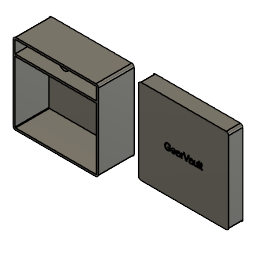
GearVault_Mini (Autodesk Fusion 360 design; units mm, degrees)
part number: 2026-09-08-22-04-46-192
Autodesk Fusion 360 part; units mm, degrees
sketch "Sketch1" plane through (0, 0, 0) normal (0, 0, 1) x (1, 0, 0)
  line L0 (-34.5, -32.5) -> (34.5, -32.5)
  line L1 (34.5, -32.5) -> (34.5, 32.5)
  line L2 (34.5, 32.5) -> (-34.5, 32.5)
  line L3 (-34.5, 32.5) -> (-34.5, -32.5)
extrude "Extrude1" add sketch "Sketch1" along normal blind 29 makes body 1
fillet "Fillet1" radius 2 4 edges at (-34.5, 32.5, 14.5) (34.5, 32.5, 14.5) (34.5, -32.5, 14.5) (-34.5, -32.5, 14.5) on bodies 1
shell "Shell1" thickness 1.6 removed faces 1 at (-10.8333, -10.8333, 29) on bodies 1
sketch "Sketch2" plane through (0, 0, 0) normal (0, 0, 1) x (1, 0, 0)
  line L0 (-32.9, 19.1) -> (32.9, 19.1)
  line L1 (32.9, 19.1) -> (32.9, 20.7)
  line L2 (32.9, 20.7) -> (-32.9, 20.7)
  line L3 (-32.9, 20.7) -> (-32.9, 19.1)
extrude "Extrude2" add sketch "Sketch2" along normal blind 29 bodies 1
sketch "Sketch3" plane through (0, 0, 0) normal (0, 0, 1) x (1, 0, 0)
  circle A0 centre (0, 25.8) radius 4
extrude "Extrude3" add sketch "Sketch3" along normal blind 22 bodies 1
sketch "Sketch4" plane through (0, 0, 0) normal (0, 0, 1) x (1, 0, 0)
  line L0 (49.5, -34.4) -> (122.3, -34.4)
  line L1 (122.3, -34.4) -> (122.3, 34.4)
  line L2 (122.3, 34.4) -> (49.5, 34.4)
  line L3 (49.5, 34.4) -> (49.5, -34.4)
sketch "Sketch6" plane through (0, 0, 0) normal (0, 0, 1) x (1, 0, 0)
  line L0 (49.5, -34.4) -> (122.3, -34.4)
  line L1 (122.3, -34.4) -> (122.3, 34.4)
  line L2 (122.3, 34.4) -> (49.5, 34.4)
  line L3 (49.5, 34.4) -> (49.5, -34.4)
extrude "Extrude6" add sketch "Sketch6" along normal blind 11.6 separate body makes body 2
fillet "Fillet3" radius 2 4 edges at (49.5, 34.4, 5.8) (122.3, 34.4, 5.8) (122.3, -34.4, 5.8) (49.5, -34.4, 5.8) on bodies 2
shell "Shell3" thickness 1.6 removed faces 1 at (74.4333, -11.4667, 0) on bodies 2
sketch "Sketch9" plane through (0, 0, 11.6) normal (0, 0, 1) x (1, 0, 0)
  arc A0 (49.5, -32.4) -> (51.5, -34.4) centre (51.5, -32.4) ccw
  line L0 (51.5, -34.4) -> (120.3, -34.4)
  arc A1 (120.3, -34.4) -> (122.3, -32.4) centre (120.3, -32.4) ccw
  line L1 (122.3, -32.4) -> (122.3, 32.4)
  arc A2 (122.3, 32.4) -> (120.3, 34.4) centre (120.3, 32.4) ccw
  line L2 (120.3, 34.4) -> (51.5, 34.4)
  arc A3 (51.5, 34.4) -> (49.5, 32.4) centre (51.5, 32.4) ccw
  line L3 (49.5, 32.4) -> (49.5, -32.4)
  line L4 (73.1527, -0.5389) -> (73.1527, 0.0477)
  line L5 (73.1527, 0.0477) -> (75.2707, 0.0512)
  line L6 (75.2707, 0.0512) -> (75.2707, -1.8042)
  spline S0 degree 2 poles (75.2707, -1.8042) (74.783, -2.193) (74.2646, -2.3892) knots 0 0 0 1 1 1
  spline S1 degree 2 poles (74.2646, -2.3892) (73.7462, -2.5853) (73.2005, -2.5853) knots 0 0 0 1 1 1
  spline S2 degree 2 poles (73.2005, -2.5853) (72.4638, -2.5853) (71.8618, -2.2698) knots 0 0 0 1 1 1
  spline S3 degree 2 poles (71.8618, -2.2698) (71.2598, -1.9543) (70.9529, -1.3574) knots 0 0 0 1 1 1
  spline S4 degree 2 poles (70.9529, -1.3574) (70.6459, -0.7606) (70.6459, -0.0239) knots 0 0 0 1 1 1
  spline S5 degree 2 poles (70.6459, -0.0239) (70.6459, 0.706) (70.9512, 1.3387) knots 0 0 0 1 1 1
  spline S6 degree 2 poles (70.9512, 1.3387) (71.2564, 1.9714) (71.8294, 2.2783) knots 0 0 0 1 1 1
  spline S7 degree 2 poles (71.8294, 2.2783) (72.4024, 2.5853) (73.1493, 2.5853) knots 0 0 0 1 1 1
  spline S8 degree 2 poles (73.1493, 2.5853) (73.6916, 2.5853) (74.1299, 2.4096) knots 0 0 0 1 1 1
  spline S9 degree 2 poles (74.1299, 2.4096) (74.5681, 2.234) (74.8171, 1.9202) knots 0 0 0 1 1 1
  spline S10 degree 2 poles (74.8171, 1.9202) (75.0661, 1.6064) (75.1957, 1.1016) knots 0 0 0 1 1 1
  line L7 (75.1957, 1.1016) -> (74.5988, 0.9379)
  spline S11 degree 2 poles (74.5988, 0.9379) (74.4863, 1.3199) (74.3192, 1.5382) knots 0 0 0 1 1 1
  spline S12 degree 2 poles (74.3192, 1.5382) (74.152, 1.7565) (73.8417, 1.8878) knots 0 0 0 1 1 1
  spline S13 degree 2 poles (73.8417, 1.8878) (73.5313, 2.0191) (73.1527, 2.0191) knots 0 0 0 1 1 1
  spline S14 degree 2 poles (73.1527, 2.0191) (72.6991, 2.0191) (72.3683, 1.881) knots 0 0 0 1 1 1
  spline S15 degree 2 poles (72.3683, 1.881) (72.0374, 1.7428) (71.8345, 1.5177) knots 0 0 0 1 1 1
  spline S16 degree 2 poles (71.8345, 1.5177) (71.6316, 1.2926) (71.519, 1.0232) knots 0 0 0 1 1 1
  spline S17 degree 2 poles (71.519, 1.0232) (71.328, 0.5593) (71.328, 0.0171) knots 0 0 0 1 1 1
  spline S18 degree 2 poles (71.328, 0.0171) (71.328, -0.6514) (71.5583, -1.1016) knots 0 0 0 1 1 1
  spline S19 degree 2 poles (71.5583, -1.1016) (71.7885, -1.5518) (72.2284, -1.7701) knots 0 0 0 1 1 1
  spline S20 degree 2 poles (72.2284, -1.7701) (72.6684, -1.9884) (73.163, -1.9884) knots 0 0 0 1 1 1
  spline S21 degree 2 poles (73.163, -1.9884) (73.5927, -1.9884) (74.002, -1.823) knots 0 0 0 1 1 1
  spline S22 degree 2 poles (74.002, -1.823) (74.4113, -1.6576) (74.6227, -1.47) knots 0 0 0 1 1 1
  line L8 (74.6227, -1.47) -> (74.6227, -0.5389)
  line L9 (74.6227, -0.5389) -> (73.1527, -0.5389)
  line L10 (78.6473, -1.3336) -> (79.2817, -1.412)
  spline S23 degree 2 poles (79.2817, -1.412) (79.1316, -1.9679) (78.7257, -2.2749) knots 0 0 0 1 1 1
  spline S24 degree 2 poles (78.7257, -2.2749) (78.3199, -2.5819) (77.6889, -2.5819) knots 0 0 0 1 1 1
  spline S25 degree 2 poles (77.6889, -2.5819) (76.8942, -2.5819) (76.4286, -2.0924) knots 0 0 0 1 1 1
  spline S26 degree 2 poles (76.4286, -2.0924) (75.9631, -1.603) (75.9631, -0.7196) knots 0 0 0 1 1 1
  spline S27 degree 2 poles (75.9631, -0.7196) (75.9631, 0.1944) (76.4338, 0.6992) knots 0 0 0 1 1 1
  spline S28 degree 2 poles (76.4338, 0.6992) (76.9044, 1.204) (77.6548, 1.204) knots 0 0 0 1 1 1
  spline S29 degree 2 poles (77.6548, 1.204) (78.3812, 1.204) (78.8417, 0.7094) knots 0 0 0 1 1 1
  spline S30 degree 2 poles (78.8417, 0.7094) (79.3021, 0.2149) (79.3021, -0.6821) knots 0 0 0 1 1 1
  spline S31 degree 2 poles (79.3021, -0.6821) (79.3021, -0.7367) (79.2987, -0.8458) knots 0 0 0 1 1 1
  line L11 (79.2987, -0.8458) -> (76.5975, -0.8458)
  spline S32 degree 2 poles (76.5975, -0.8458) (76.6316, -1.4427) (76.9351, -1.7599) knots 0 0 0 1 1 1
  spline S33 degree 2 poles (76.9351, -1.7599) (77.2387, -2.0771) (77.6923, -2.0771) knots 0 0 0 1 1 1
  spline S34 degree 2 poles (77.6923, -2.0771) (78.0299, -2.0771) (78.2687, -1.8997) knots 0 0 0 1 1 1
  spline S35 degree 2 poles (78.2687, -1.8997) (78.5074, -1.7224) (78.6473, -1.3336) knots 0 0 0 1 1 1
  line L12 (76.6316, -0.3411) -> (78.6541, -0.3411)
  spline S36 degree 2 poles (78.6541, -0.3411) (78.6132, 0.116) (78.4222, 0.3445) knots 0 0 0 1 1 1
  spline S37 degree 2 poles (78.4222, 0.3445) (78.1289, 0.6992) (77.6616, 0.6992) knots 0 0 0 1 1 1
  spline S38 degree 2 poles (77.6616, 0.6992) (77.2387, 0.6992) (76.9505, 0.4161) knots 0 0 0 1 1 1
  spline S39 degree 2 poles (76.9505, 0.4161) (76.6623, 0.133) (76.6316, -0.3411) knots 0 0 0 1 1 1
  spline S40 degree 2 poles (82.416, -2.0532) (82.075, -2.3431) (81.7595, -2.4625) knots 0 0 0 1 1 1
  spline S41 degree 2 poles (81.7595, -2.4625) (81.444, -2.5819) (81.0825, -2.5819) knots 0 0 0 1 1 1
  spline S42 degree 2 poles (81.0825, -2.5819) (80.4856, -2.5819) (80.165, -2.2902) knots 0 0 0 1 1 1
  spline S43 degree 2 poles (80.165, -2.2902) (79.8444, -1.9986) (79.8444, -1.545) knots 0 0 0 1 1 1
  spline S44 degree 2 poles (79.8444, -1.545) (79.8444, -1.279) (79.9655, -1.059) knots 0 0 0 1 1 1
  spline S45 degree 2 poles (79.9655, -1.059) (80.0866, -0.839) (80.2827, -0.706) knots 0 0 0 1 1 1
  spline S46 degree 2 poles (80.2827, -0.706) (80.4788, -0.573) (80.7244, -0.5048) knots 0 0 0 1 1 1
  spline S47 degree 2 poles (80.7244, -0.5048) (80.9051, -0.457) (81.2701, -0.4127) knots 0 0 0 1 1 1
  spline S48 degree 2 poles (81.2701, -0.4127) (82.0136, -0.324) (82.3649, -0.2012) knots 0 0 0 1 1 1
  spline S49 degree 2 poles (82.3649, -0.2012) (82.3683, -0.075) (82.3683, -0.0409) knots 0 0 0 1 1 1
  spline S50 degree 2 poles (82.3683, -0.0409) (82.3683, 0.3342) (82.1943, 0.4877) knots 0 0 0 1 1 1
  spline S51 degree 2 poles (82.1943, 0.4877) (81.959, 0.6958) (81.4952, 0.6958) knots 0 0 0 1 1 1
  spline S52 degree 2 poles (81.4952, 0.6958) (81.062, 0.6958) (80.8557, 0.544) knots 0 0 0 1 1 1
  spline S53 degree 2 poles (80.8557, 0.544) (80.6493, 0.3922) (80.5504, 0.0068) knots 0 0 0 1 1 1
  line L13 (80.5504, 0.0068) -> (79.9501, 0.0887)
  spline S54 degree 2 poles (79.9501, 0.0887) (80.032, 0.4741) (80.2196, 0.7111) knots 0 0 0 1 1 1
  spline S55 degree 2 poles (80.2196, 0.7111) (80.4072, 0.9482) (80.7619, 1.0761) knots 0 0 0 1 1 1
  spline S56 degree 2 poles (80.7619, 1.0761) (81.1166, 1.204) (81.5838, 1.204) knots 0 0 0 1 1 1
  spline S57 degree 2 poles (81.5838, 1.204) (82.0477, 1.204) (82.3376, 1.0948) knots 0 0 0 1 1 1
  spline S58 degree 2 poles (82.3376, 1.0948) (82.6275, 0.9857) (82.7639, 0.8203) knots 0 0 0 1 1 1
  spline S59 degree 2 poles (82.7639, 0.8203) (82.9003, 0.6548) (82.9549, 0.4025) knots 0 0 0 1 1 1
  spline S60 degree 2 poles (82.9549, 0.4025) (82.9856, 0.2456) (82.9856, -0.1637) knots 0 0 0 1 1 1
  line L14 (82.9856, -0.1637) -> (82.9856, -0.9823)
  spline S61 degree 2 poles (82.9856, -0.9823) (82.9856, -1.8383) (83.0248, -2.0651) knots 0 0 0 1 1 1
  spline S62 degree 2 poles (83.0248, -2.0651) (83.0641, -2.292) (83.18, -2.5) knots 0 0 0 1 1 1
  line L15 (83.18, -2.5) -> (82.5388, -2.5)
  spline S63 degree 2 poles (82.5388, -2.5) (82.4433, -2.309) (82.416, -2.0532) knots 0 0 0 1 1 1
  spline S64 degree 2 poles (82.3649, -0.6821) (82.0306, -0.8186) (81.3621, -0.9141) knots 0 0 0 1 1 1
  spline S65 degree 2 poles (81.3621, -0.9141) (80.9836, -0.9686) (80.8267, -1.0368) knots 0 0 0 1 1 1
  spline S66 degree 2 poles (80.8267, -1.0368) (80.6698, -1.105) (80.5845, -1.2364) knots 0 0 0 1 1 1
  spline S67 degree 2 poles (80.5845, -1.2364) (80.4992, -1.3677) (80.4992, -1.528) knots 0 0 0 1 1 1
  spline S68 degree 2 poles (80.4992, -1.528) (80.4992, -1.7735) (80.6851, -1.9372) knots 0 0 0 1 1 1
  spline S69 degree 2 poles (80.6851, -1.9372) (80.871, -2.101) (81.2291, -2.101) knots 0 0 0 1 1 1
  spline S70 degree 2 poles (81.2291, -2.101) (81.5838, -2.101) (81.8601, -1.9458) knots 0 0 0 1 1 1
  spline S71 degree 2 poles (81.8601, -1.9458) (82.1364, -1.7906) (82.266, -1.5211) knots 0 0 0 1 1 1
  spline S72 degree 2 poles (82.266, -1.5211) (82.3649, -1.3131) (82.3649, -0.9072) knots 0 0 0 1 1 1
  line L16 (82.3649, -0.9072) -> (82.3649, -0.6821)
  line L17 (83.9304, -2.5) -> (83.9304, 1.1221)
  line L18 (83.9304, 1.1221) -> (84.4829, 1.1221)
  line L19 (84.4829, 1.1221) -> (84.4829, 0.573)
  spline S73 degree 2 poles (84.4829, 0.573) (84.6943, 0.9584) (84.8734, 1.0812) knots 0 0 0 1 1 1
  spline S74 degree 2 poles (84.8734, 1.0812) (85.0525, 1.204) (85.2673, 1.204) knots 0 0 0 1 1 1
  spline S75 degree 2 poles (85.2673, 1.204) (85.5777, 1.204) (85.8983, 1.0061) knots 0 0 0 1 1 1
  line L20 (85.8983, 1.0061) -> (85.6868, 0.4366)
  spline S76 degree 2 poles (85.6868, 0.4366) (85.4617, 0.5696) (85.2366, 0.5696) knots 0 0 0 1 1 1
  spline S77 degree 2 poles (85.2366, 0.5696) (85.0354, 0.5696) (84.8751, 0.4485) knots 0 0 0 1 1 1
  spline S78 degree 2 poles (84.8751, 0.4485) (84.7148, 0.3274) (84.6466, 0.1126) knots 0 0 0 1 1 1
  spline S79 degree 2 poles (84.6466, 0.1126) (84.5443, -0.2149) (84.5443, -0.6037) knots 0 0 0 1 1 1
  line L21 (84.5443, -0.6037) -> (84.5443, -2.5)
  line L22 (84.5443, -2.5) -> (83.9304, -2.5)
  line L23 (87.7707, -2.5) -> (85.8335, 2.5)
  line L24 (85.8335, 2.5) -> (86.5497, 2.5)
  line L25 (86.5497, 2.5) -> (87.8492, -1.1323)
  spline S80 degree 2 poles (87.8492, -1.1323) (88.0061, -1.5689) (88.1118, -1.9509) knots 0 0 0 1 1 1
  spline S81 degree 2 poles (88.1118, -1.9509) (88.2278, -1.5416) (88.3812, -1.1323) knots 0 0 0 1 1 1
  line L26 (88.3812, -1.1323) -> (89.7319, 2.5)
  line L27 (89.7319, 2.5) -> (90.4072, 2.5)
  line L28 (90.4072, 2.5) -> (88.4495, -2.5)
  line L29 (88.4495, -2.5) -> (87.7707, -2.5)
  spline S82 degree 2 poles (92.7673, -2.0532) (92.4263, -2.3431) (92.1108, -2.4625) knots 0 0 0 1 1 1
  spline S83 degree 2 poles (92.1108, -2.4625) (91.7953, -2.5819) (91.4338, -2.5819) knots 0 0 0 1 1 1
  spline S84 degree 2 poles (91.4338, -2.5819) (90.8369, -2.5819) (90.5163, -2.2902) knots 0 0 0 1 1 1
  spline S85 degree 2 poles (90.5163, -2.2902) (90.1957, -1.9986) (90.1957, -1.545) knots 0 0 0 1 1 1
  spline S86 degree 2 poles (90.1957, -1.545) (90.1957, -1.279) (90.3168, -1.059) knots 0 0 0 1 1 1
  spline S87 degree 2 poles (90.3168, -1.059) (90.4379, -0.839) (90.634, -0.706) knots 0 0 0 1 1 1
  spline S88 degree 2 poles (90.634, -0.706) (90.8301, -0.573) (91.0756, -0.5048) knots 0 0 0 1 1 1
  spline S89 degree 2 poles (91.0756, -0.5048) (91.2564, -0.457) (91.6214, -0.4127) knots 0 0 0 1 1 1
  spline S90 degree 2 poles (91.6214, -0.4127) (92.3649, -0.324) (92.7162, -0.2012) knots 0 0 0 1 1 1
  spline S91 degree 2 poles (92.7162, -0.2012) (92.7196, -0.075) (92.7196, -0.0409) knots 0 0 0 1 1 1
  spline S92 degree 2 poles (92.7196, -0.0409) (92.7196, 0.3342) (92.5456, 0.4877) knots 0 0 0 1 1 1
  spline S93 degree 2 poles (92.5456, 0.4877) (92.3103, 0.6958) (91.8465, 0.6958) knots 0 0 0 1 1 1
  spline S94 degree 2 poles (91.8465, 0.6958) (91.4133, 0.6958) (91.207, 0.544) knots 0 0 0 1 1 1
  spline S95 degree 2 poles (91.207, 0.544) (91.0006, 0.3922) (90.9017, 0.0068) knots 0 0 0 1 1 1
  line L30 (90.9017, 0.0068) -> (90.3014, 0.0887)
  spline S96 degree 2 poles (90.3014, 0.0887) (90.3833, 0.4741) (90.5709, 0.7111) knots 0 0 0 1 1 1
  spline S97 degree 2 poles (90.5709, 0.7111) (90.7585, 0.9482) (91.1132, 1.0761) knots 0 0 0 1 1 1
  spline S98 degree 2 poles (91.1132, 1.0761) (91.4679, 1.204) (91.9351, 1.204) knots 0 0 0 1 1 1
  spline S99 degree 2 poles (91.9351, 1.204) (92.399, 1.204) (92.6889, 1.0948) knots 0 0 0 1 1 1
  spline S100 degree 2 poles (92.6889, 1.0948) (92.9788, 0.9857) (93.1152, 0.8203) knots 0 0 0 1 1 1
  spline S101 degree 2 poles (93.1152, 0.8203) (93.2516, 0.6548) (93.3062, 0.4025) knots 0 0 0 1 1 1
  spline S102 degree 2 poles (93.3062, 0.4025) (93.3369, 0.2456) (93.3369, -0.1637) knots 0 0 0 1 1 1
  line L31 (93.3369, -0.1637) -> (93.3369, -0.9823)
  spline S103 degree 2 poles (93.3369, -0.9823) (93.3369, -1.8383) (93.3761, -2.0651) knots 0 0 0 1 1 1
  spline S104 degree 2 poles (93.3761, -2.0651) (93.4153, -2.292) (93.5313, -2.5) knots 0 0 0 1 1 1
  line L32 (93.5313, -2.5) -> (92.8901, -2.5)
  spline S105 degree 2 poles (92.8901, -2.5) (92.7946, -2.309) (92.7673, -2.0532) knots 0 0 0 1 1 1
  spline S106 degree 2 poles (92.7162, -0.6821) (92.3819, -0.8186) (91.7134, -0.9141) knots 0 0 0 1 1 1
  spline S107 degree 2 poles (91.7134, -0.9141) (91.3349, -0.9686) (91.178, -1.0368) knots 0 0 0 1 1 1
  spline S108 degree 2 poles (91.178, -1.0368) (91.0211, -1.105) (90.9358, -1.2364) knots 0 0 0 1 1 1
  spline S109 degree 2 poles (90.9358, -1.2364) (90.8505, -1.3677) (90.8505, -1.528) knots 0 0 0 1 1 1
  spline S110 degree 2 poles (90.8505, -1.528) (90.8505, -1.7735) (91.0364, -1.9372) knots 0 0 0 1 1 1
  spline S111 degree 2 poles (91.0364, -1.9372) (91.2223, -2.101) (91.5804, -2.101) knots 0 0 0 1 1 1
  spline S112 degree 2 poles (91.5804, -2.101) (91.9351, -2.101) (92.2114, -1.9458) knots 0 0 0 1 1 1
  spline S113 degree 2 poles (92.2114, -1.9458) (92.4877, -1.7906) (92.6173, -1.5211) knots 0 0 0 1 1 1
  spline S114 degree 2 poles (92.6173, -1.5211) (92.7162, -1.3131) (92.7162, -0.9072) knots 0 0 0 1 1 1
  line L33 (92.7162, -0.9072) -> (92.7162, -0.6821)
  line L34 (96.6623, -2.5) -> (96.6623, -1.9679)
  spline S115 degree 2 poles (96.6623, -1.9679) (96.2394, -2.5819) (95.5129, -2.5819) knots 0 0 0 1 1 1
  spline S116 degree 2 poles (95.5129, -2.5819) (95.1923, -2.5819) (94.9143, -2.4591) knots 0 0 0 1 1 1
  spline S117 degree 2 poles (94.9143, -2.4591) (94.6364, -2.3363) (94.5016, -2.1504) knots 0 0 0 1 1 1
  spline S118 degree 2 poles (94.5016, -2.1504) (94.3669, -1.9645) (94.3123, -1.6951) knots 0 0 0 1 1 1
  spline S119 degree 2 poles (94.3123, -1.6951) (94.2748, -1.5143) (94.2748, -1.1221) knots 0 0 0 1 1 1
  line L35 (94.2748, -1.1221) -> (94.2748, 1.1221)
  line L36 (94.2748, 1.1221) -> (94.8887, 1.1221)
  line L37 (94.8887, 1.1221) -> (94.8887, -0.8868)
  spline S120 degree 2 poles (94.8887, -0.8868) (94.8887, -1.3677) (94.9263, -1.5348) knots 0 0 0 1 1 1
  spline S121 degree 2 poles (94.9263, -1.5348) (94.9842, -1.7769) (95.1718, -1.9151) knots 0 0 0 1 1 1
  spline S122 degree 2 poles (95.1718, -1.9151) (95.3594, -2.0532) (95.6357, -2.0532) knots 0 0 0 1 1 1
  spline S123 degree 2 poles (95.6357, -2.0532) (95.9119, -2.0532) (96.1541, -1.9117) knots 0 0 0 1 1 1
  spline S124 degree 2 poles (96.1541, -1.9117) (96.3962, -1.7701) (96.4969, -1.5263) knots 0 0 0 1 1 1
  spline S125 degree 2 poles (96.4969, -1.5263) (96.5975, -1.2824) (96.5975, -0.8186) knots 0 0 0 1 1 1
  line L38 (96.5975, -0.8186) -> (96.5975, 1.1221)
  line L39 (96.5975, 1.1221) -> (97.2114, 1.1221)
  line L40 (97.2114, 1.1221) -> (97.2114, -2.5)
  line L41 (97.2114, -2.5) -> (96.6623, -2.5)
  line L42 (98.1596, -2.5) -> (98.1596, 2.5)
  line L43 (98.1596, 2.5) -> (98.7735, 2.5)
  line L44 (98.7735, 2.5) -> (98.7735, -2.5)
  line L45 (98.7735, -2.5) -> (98.1596, -2.5)
  line L46 (101.0654, -1.9509) -> (101.1541, -2.4932)
  spline S126 degree 2 poles (101.1541, -2.4932) (100.8949, -2.5477) (100.6902, -2.5477) knots 0 0 0 1 1 1
  spline S127 degree 2 poles (100.6902, -2.5477) (100.356, -2.5477) (100.1718, -2.442) knots 0 0 0 1 1 1
  spline S128 degree 2 poles (100.1718, -2.442) (99.9877, -2.3363) (99.9126, -2.1641) knots 0 0 0 1 1 1
  spline S129 degree 2 poles (99.9126, -2.1641) (99.8376, -1.9918) (99.8376, -1.4393) knots 0 0 0 1 1 1
  line L47 (99.8376, -1.4393) -> (99.8376, 0.6446)
  line L48 (99.8376, 0.6446) -> (99.3874, 0.6446)
  line L49 (99.3874, 0.6446) -> (99.3874, 1.1221)
  line L50 (99.3874, 1.1221) -> (99.8376, 1.1221)
  line L51 (99.8376, 1.1221) -> (99.8376, 2.0191)
  line L52 (99.8376, 2.0191) -> (100.4481, 2.3874)
  line L53 (100.4481, 2.3874) -> (100.4481, 1.1221)
  line L54 (100.4481, 1.1221) -> (101.0654, 1.1221)
  line L55 (101.0654, 1.1221) -> (101.0654, 0.6446)
  line L56 (101.0654, 0.6446) -> (100.4481, 0.6446)
  line L57 (100.4481, 0.6446) -> (100.4481, -1.4734)
  spline S130 degree 2 poles (100.4481, -1.4734) (100.4481, -1.736) (100.4805, -1.8111) knots 0 0 0 1 1 1
  spline S131 degree 2 poles (100.4805, -1.8111) (100.5129, -1.8861) (100.5862, -1.9304) knots 0 0 0 1 1 1
  spline S132 degree 2 poles (100.5862, -1.9304) (100.6595, -1.9748) (100.796, -1.9748) knots 0 0 0 1 1 1
  spline S133 degree 2 poles (100.796, -1.9748) (100.8983, -1.9748) (101.0654, -1.9509) knots 0 0 0 1 1 1
extrude "Extrude9" cut sketch "Sketch9" against normal blind 0.4 contours L4 L5 L6 S0 S1 S2 S3 S4 S5 S6 S7 S8 S9 S10 L7 S11 S12 S13 S14 S15 S16 S17 S18 S19 S20 S21 S22 L8 L9 | L10 S23 S24 S25 S26 S27 S28 S29 S30 S31 L11 S32 S33 S34 S35 | L12 S36 S37 S38 S39 | S40 S41 S42 S43 S44 S45 S46 S47 S48 S49 S50 S51 S52 S53 L13 S54 S55 S56 S57 S58 S59 S60 L14 S61 S62 L15 S63 | S64 S65 S66 S67 S68 S69 S70 S71 S72 L16 | L17 L18 L19 S73 S74 S75 L20 S76 S77 S78 S79 L21 L22 | L23 L24 L25 S80 S81 L26 L27 L28 L29 | S82 S83 S84 S85 S86 S87 S88 S89 S90 S91 S92 S93 S94 S95 L30 S96 S97 S98 S99 S100 S101 S102 L31 S103 S104 L32 S105 | S106 S107 S108 S109 S110 S111 S112 S113 S114 L33 | L34 S115 S116 S117 S118 S119 L35 L36 L37 S120 S121 S122 S123 S124 S125 L38 L39 L40 L41 | L42 L43 L44 L45 | L46 S126 S127 S128 S129 L47 L48 L49 L50 L51 L52 L53 L54 L55 L56 L57 S130 S131 S132 S133 bodies 2
named bodies: "Base", "Lid"
